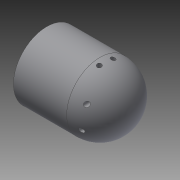
# Autodesk Inventor part: pressure-end
Saved by Autodesk Inventor 2014 SP2 (Build 180246200, 246)
## iProperties
Created: 2014-06-30
Part Number: pressure-end
Material: Generic
Document SubType Name: Modeling
Designer: pjb08r
Density: 1 g/cm^3
Appearance: Default
Author: pjb08r
Autodesk Inventor part; units mm, degrees
ref_plane "YZ Plane" through (0, 0, 0) normal (1, 0, 0) x (0, 1, 0)
ref_plane "XZ Plane" through (0, 0, 0) normal (0, 1, 0) x (-1, 0, 0)
ref_plane "XY Plane" through (0, 0, 0) normal (0, 0, 1) x (1, 0, 0)
sketch "Sketch1" plane through (0, 0, 0) normal (1, 0, 0) x (0, 1, 0)
  circle A0 centre (0, 0) radius 7.5
  dimension "d0" = 15
  constraints: 1 centre point, 1 coincident
  measures "d0" diameter of A0
extrude "Extrusion1" add sketch "Sketch1" along normal blind 12
hole "Hole1" at (12, -0.0383, -0.034) direction (-1, 0, 0) diameter 9.728 end through all thread size "7/16-20 UNF" class "2B" standard "ANSI Unified Screw Threads"
sketch "Sketch2" plane through (12, 0, 0) normal (1, 0, 0) x (0, 0, -1)
  circle A0 centre (0, 0) radius 7.5 projected
  circle A1 centre (0, 0) radius 7.5
  constraints: 1 centre point, 1 coincident, 1 concentric
extrude "Extrusion2" add sketch "Sketch2" along normal blind 7.5
ref_plane "Work Plane1" through (15, -0.0383, -0.034) normal (-1, 0, 0) x (0, 0, 1)
sketch "Sketch3" plane through (12, -0.0383, -0.034) normal (-1, 0, 0) x (0, 0, 1)
  line L0 (-3, -3) -> (3.6, -3)
  line L1 (3.6, -3) -> (3.6, 2.703)
  line L2 (3.6, 2.703) -> (-3, 2.703)
  line L3 (-3, 2.703) -> (-3, -3)
  point P0 (0.034, 0.0383)
  dimension "d26" = 6.6
  constraints: 8 end point, 2 parallel, 1 horizontal, 1 perpendicular
  measures "d26" distance of L2.end L1.end
extrude "Extrusion3" cut sketch "Sketch3" against normal blind 4
fillet "Fillet2" radius 7.5 1 edges at (19.5, 0, 7.5)
hole "Hole3" at (13.8552, 2.6647, 2.5355) direction (0, 1, 0) diameter 1 end through all
hole "Hole4" at (13.6818, 2.6647, -1.978) direction (0, 1, 0) diameter 1 end through all
hole "Hole5" at (13.4458, 1.4998, 3.566) direction (0, 0, 1) diameter 1 end through all
hole "Hole6" at (13.2606, -1.4148, 3.566) direction (0, 0, 1) diameter 1 end through all
hole "Hole7" at (15.1514, -3.0383, 2.9639) direction (0, -1, 0) diameter 1 end through all
hole "Hole8" at (13.8338, 1.4837, -3.034) direction (0, 0, -1) diameter 1 end through all
hole "Hole9" at (14.5992, -3.0383, -2.132) direction (0, -1, 0) diameter 1 end through all
hole "Hole10" at (14.224, -2.0448, -3.034) direction (0, 0, -1) diameter 1 end through all
body "Solid1"
